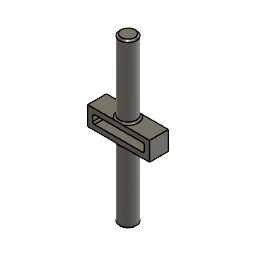
Pilar camara V3 (Autodesk Fusion 360 design; units mm, degrees)
Autodesk Fusion 360 part; units mm, degrees
sketch "Sketch1" plane through (0, 0, 0) normal (0, 0, 1) x (1, 0, 0)
  line L0 (-15, 2.5) -> (15, 2.5)
  line L1 (15, 2.5) -> (15, -2.5)
  line L2 (15, -2.5) -> (-15, -2.5)
  line L3 (-15, -2.5) -> (-15, 2.5)
  line L4 (-15, 2.5) -> (15, -2.5) construction
  line L5 (15, 2.5) -> (-15, -2.5) construction
  line L6 (18, -5.5) -> (-18, -5.5)
  line L7 (-18, -5.5) -> (-18, 5.5)
  line L8 (-18, 5.5) -> (18, 5.5)
  line L9 (18, 5.5) -> (18, -5.5)
  dimension "d1" = 30
  dimension "d2" = 5
  dimension "d4" = -3
  constraint horizontal L0
  constraint perpendicular L0 L1
  constraint parallel L0 L2
  constraint parallel L1 L3
  constraint coincident L4 origin
  constraint coincident L5 origin
  measures "d1" distance of L1 L3
  measures "d2" distance of L0.end L1.end
extrude "Extrude1" add sketch "Sketch1" against normal blind 11
sketch "Sketch2" plane through (0, 5.5, 0) normal (0, 1, 0) x (-1, 0, 0)
  line L0 (18, 0) -> (-18, 0)
  line L1 (-18, 0) -> (-18, -11)
  line L2 (-18, -11) -> (18, -11)
  line L3 (18, -11) -> (18, 0)
  circle A0 centre (0, -5.5) radius 5
  dimension "d11" = 5.5
  measures "d11" distance of L2 A0.centre
extrude "Extrude2" add sketch "Sketch2" along normal blind 42 contours A0
mirror "Mirror1" about plane through (0, 0, 0) normal (0, 1, 0) of bodies 1 merged
fillet "Fillet1" radius 1 2 edges at (4.6616, 5.5, -3.6919) (4.6616, -5.5, -7.3081)
chamfer "Chamfer1" distance 1 angle 45 2 edges at (4.6616, 47.5, -7.3081) (4.6616, -47.5, -7.3081)
fillet "Fillet2" radius 1 4 edges at (-15, 2.5, -5.5) (-15, -2.5, -5.5) (15, -2.5, -5.5) (15, 2.5, -5.5)
